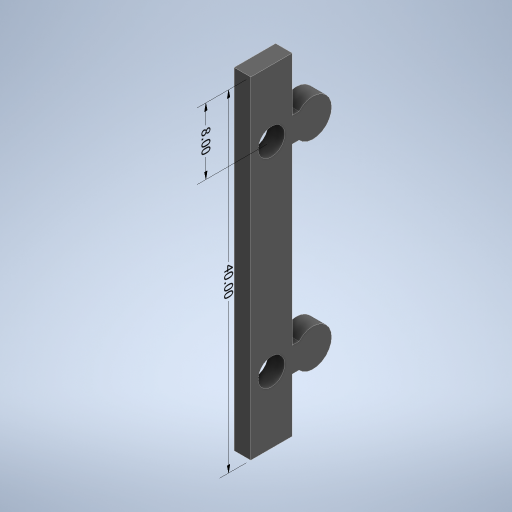
# Autodesk Inventor part: cover_setter
Saved by Autodesk Inventor 2024.1 (Build 281209000, 209)
## iProperties
Created: 2025-03-07
Part Number: cover_setter
Material: 一般
Document SubType Name: Modeling
Designer: hibik
Density: 1 g/cm^3
Appearance: 既定
Author: hibik
Autodesk Inventor part; units mm, degrees
ref_plane "YZ Plane" through (0, 0, 0) normal (1, 0, 0) x (0, 1, 0)
ref_plane "XZ Plane" through (0, 0, 0) normal (0, 1, 0) x (-1, 0, 0)
ref_plane "XY Plane" through (0, 0, 0) normal (0, 0, 1) x (1, 0, 0)
sketch "スケッチ1" plane through (0, 0, 0) normal (1, 0, 0) x (0, 1, 0)
  line L0 (20, 0) -> (0, 0)
  line L1 (0, 0) -> (0, -5)
  line L2 (0, -5) -> (20, -5)
  line L3 (20, -5) -> (20, 0)
  circle A0 centre (12, -7.5) radius 2.5 construction
  circle A1 centre (12, -7.5) radius 2.25
  line L4 (13.5, -5.8229) -> (10.5, -5.8229)
  line L5 (10.5, -5.8229) -> (10.5, -5)
  line L6 (10.5, -5) -> (13.5, -5)
  line L7 (13.5, -5) -> (13.5, -5.8229)
  line L8 (12, -7.5) -> (12, -5)
  dimension "d1" = 4.5
  dimension "d0" = 5
  dimension "d2" = 3
  dimension "d3" = 12
  dimension "d4" = 5
  dimension "d5" = 20
  constraints: 18 end point, 4 parallel, 3 perpendicular, 2 horizontal, 2 point on line, 1 centre point, 1 coincident, 1 collinear, 1 midpoint, 1 tangent, 4 other
  measures "d0" diameter of A0
  measures "d2" distance of L5.end L6.end
  measures "d3" horizontal distance of point (0, 0) A0.centre
  measures "d4" distance of L2.end L0.start
  measures "d5" distance of L0.start L0.end
extrude "押し出し1" add sketch "スケッチ1" along normal blind 2
mirror "ミラー1" about plane through (0, 0, 0) normal (0, -1, 0)
sketch "スケッチ2" plane through (2, 0, 0) normal (1, 0, 0) x (0, 0, -1)
  line L0 (5.8229, 13.5) -> (5, 13.5) projected
  line L1 (5, 13.5) -> (5, 20) projected
  line L2 (5, 20) -> (0, 20) projected
  line L3 (0, 20) -> (0, -20) projected
  line L4 (5, -20) -> (0, -20) projected
  line L5 (5, -13.5) -> (5, -20) projected
  line L6 (5.8229, -13.5) -> (5, -13.5) projected
  arc A0 (5.8229, -13.5) -> (5.8229, -10.5) centre (7.5, -12) ccw projected
  line L7 (5, -10.5) -> (5.8229, -10.5) projected
  line L8 (5, 10.5) -> (5, -10.5) projected
  line L9 (5, 10.5) -> (5.8229, 10.5) projected
  arc A1 (5.8229, 10.5) -> (5.8229, 13.5) centre (7.5, 12) ccw projected
  circle A2 centre (2.5, 12) radius 1.6
  circle A3 centre (2.5, -12) radius 1.6
  point P0 (0, 0)
  point P1 (2.5, 20)
  dimension "d8" = 3.2
  constraints: 2 centre point, 2 horizontal alignment, 2 vertical alignment, 1 equal radius, 1 midpoint
  measures "d8" diameter of A2
extrude "押し出し2" cut sketch "スケッチ2" against normal blind 2 contours A2 | A3
